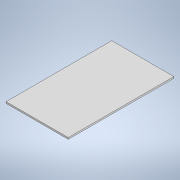
# Autodesk Inventor part: test_part_ignore
Saved by Autodesk Inventor 2021 (Build 250183000, 183)
## iProperties
Created: 2021-05-03
Part Number: test_part_ignore
Material: Generic
Document SubType Name: Modeling
Designer: ocon0143
Density: 1 g/cm^3
Appearance: Default
Author: ocon0143
Autodesk Inventor part; units mm, degrees
ref_plane "YZ Plane" through (0, 0, 0) normal (1, 0, 0) x (0, 1, 0)
ref_plane "XZ Plane" through (0, 0, 0) normal (0, 1, 0) x (-1, 0, 0)
ref_plane "XY Plane" through (0, 0, 0) normal (0, 0, 1) x (1, 0, 0)
sketch "Sketch1" plane through (0, 0, 0) normal (0, 1, 0) x (-1, 0, 0)
  line L0 (6.968, 8.0274) -> (-993.032, 8.0274)
  line L1 (-993.032, 8.0274) -> (-993.032, -1691.9726)
  line L2 (-993.032, -1691.9726) -> (6.968, -1691.9726)
  line L3 (6.968, -1691.9726) -> (6.968, 8.0274)
  point P0 (0, 0)
  dimension "d0" = 1700
  dimension "d1" = 1000
  constraints: 8 end point, 2 parallel, 1 horizontal, 1 perpendicular
  measures "d0" distance of L2.end L0.start
  measures "d1" distance of L0.start L0.end
extrude "Extrusion1" add sketch "Sketch1" along normal blind 25.4
equation "\"d0\" = testHeight"
equation "\"d1\" = testLength"
equation "\"roof_width\" = 25.4"
equation "\"testHeight\" = 1700"
equation "\"testLength\" = 1000"
body "Solid1"
